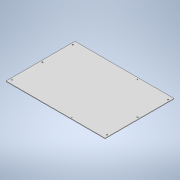
# Autodesk Inventor part: SidePanel
Saved by Autodesk Inventor 2020 (Build 240168000, 168)
## iProperties
Created: 2019-11-09
Part Number: SidePanel
Material: Generic
Document SubType Name: Modeling
Designer: nicoc
Density: 1 g/cm^3
Appearance: Default
Author: nicoc
Autodesk Inventor part; units mm, degrees
ref_plane "YZ Plane" through (0, 0, 0) normal (1, 0, 0) x (0, 1, 0)
ref_plane "XZ Plane" through (0, 0, 0) normal (0, 1, 0) x (-1, 0, 0)
ref_plane "XY Plane" through (0, 0, 0) normal (0, 0, 1) x (1, 0, 0)
sketch "Sketch1" plane through (0, 0, 0) normal (0, 1, 0) x (-1, 0, 0)
  line L0 (0, 0) -> (1000, 0)
  line L1 (1000, 0) -> (1000, -695)
  line L2 (1000, -695) -> (0, -695)
  line L3 (0, -695) -> (0, 0)
  dimension "d0" = 695
  dimension "d1" = 1000
  constraints: 8 end point, 2 parallel, 1 horizontal, 1 perpendicular
  measures "d0" distance between parallel lines of L2 L0
  measures "d1" distance between parallel lines of L1 L3
extrude "Extrusion1" add sketch "Sketch1" along normal blind 5
sketch "Sketch2" plane through (0, 5, 0) normal (0, 1, 0) x (1, 0, 0)
  line L0 (-1000, 0) -> (0, 0) projected
  line L1 (0, 0) -> (0, 695) projected
  line L2 (0, 695) -> (-1000, 695) projected
  line L3 (-1000, 695) -> (-1000, 0) projected
  point P0 (-20, 40)
  point P1 (-20, 347.5)
  point P2 (-20, 655)
  point P3 (-980, 40)
  point P4 (-980, 347.5)
  point P5 (-980, 655)
  dimension "d4" = 40
  dimension "d5" = 20
  dimension "d6" = 20
  dimension "d7" = 20
  dimension "d8" = 347.5
  dimension "d9" = 40
  dimension "d14" = 40
  dimension "d15" = 40
  dimension "d16" = 347.5
  dimension "d17" = 20
  dimension "d18" = 20
  dimension "d19" = 20
  measures "d4" distance from line of point (-20, 40) L0
  measures "d5" distance from line of point (-20, 40) L1
  measures "d6" distance from line of point (-20, 347.5) L1
  measures "d7" distance from line of point (-20, 655) L1
  measures "d8" distance from line of point (-20, 347.5) L0
  measures "d9" distance from line of L2 point (-20, 655)
  measures "d14" distance from line of L0 point (-980, 40)
  measures "d15" distance from line of point (-980, 655) L2
  measures "d16" distance from line of point (-980, 347.5) L0
  measures "d17" distance from line of L3 point (-980, 40)
  measures "d18" distance from line of L3 point (-980, 347.5)
  measures "d19" distance from line of L3 point (-980, 655)
hole "Hole1" at (-20, 5, -40) at (-20, 5, -347.5) at (-20, 5, -655) at (-980, 5, -40) at (-980, 5, -347.5) at (-980, 5, -655) direction (0, -1, 0) diameter 5.5 end through all countersink diameter 11.5 countersink angle 90
sketch "Sketch3" plane through (0, 5, 0) normal (0, 1, 0) x (1, 0, 0)
  line L0 (0, 0) -> (0, 695) projected
  line L1 (-1000, 0) -> (0, 0) projected
  line L2 (0, 695) -> (-1000, 695) projected
  point P0 (-350, 15)
  point P1 (-350, 675)
  dimension "d27" = 350
  dimension "d28" = 15
  dimension "d29" = 20
  dimension "d30" = 350
  measures "d27" distance from line of L0 point (-350, 15)
  measures "d28" distance from line of L1 point (-350, 15)
  measures "d29" distance from line of L2 point (-350, 675)
  measures "d30" distance from line of L0 point (-350, 675)
hole "Hole2" at (-350, 5, -15) at (-350, 5, -675) direction (0, -1, 0) diameter 6.647 end through all thread size "M8x1.25" class "6H" standard "ISO Metric profile"
equation "\"d6\" = d5"
equation "\"d7\" = d5"
equation "\"d9\" = d4"
equation "\"d14\" = d4"
equation "\"d15\" = d4"
equation "\"d16\" = d8"
equation "\"d17\" = d5"
equation "\"d18\" = d5"
equation "\"d19\" = d5"
equation "\"d30\" = d27"
body "Solid1"
